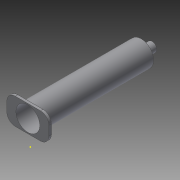
# Autodesk Inventor part: motor mount
Saved by Autodesk Inventor 2015 SP1 (Build 190203100, 203)
## iProperties
Created: 2016-07-07
Part Number: motor mount
Material: Generic
Document SubType Name: Modeling
Designer: lustinga
Density: 1 g/cm^3
Appearance: Default
Mass: 8.44804 g
Surface Area: 280.703 cm^2
Volume: 8.44804 cm^3
Author: lustinga
Autodesk Inventor part; units mm, degrees
ref_plane "YZ Plane" through (0, 0, 0) normal (1, 0, 0) x (0, 1, 0)
ref_plane "XZ Plane" through (0, 0, 0) normal (0, 1, 0) x (-1, 0, 0)
ref_plane "XY Plane" through (0, 0, 0) normal (0, 0, 1) x (1, 0, 0)
sketch "Sketch1" plane through (0, 0, 0) normal (1, 0, 0) x (0, 1, 0)
  line L0 (-81.3077, 45.4162) -> (50.6923, 45.4162)
  line L1 (56.553, 36.2588) -> (50.6923, 45.4162)
  line L2 (56.553, 36.2588) -> (63.703, 36.2588)
  line L3 (30.7678, 30.6662) -> (60.128, 30.6662)
  line L4 (63.703, 35.7588) -> (56.2794, 35.7588)
  line L5 (56.2794, 35.7588) -> (50.4187, 44.9162)
  line L6 (50.4187, 44.9162) -> (-81.3077, 44.9162)
  line L7 (63.703, 35.7588) -> (63.703, 36.2588)
  line L8 (-81.3077, 44.9162) -> (-81.3077, 45.4162)
  dimension "d26" = 132
  dimension "d29" = 7.15
  dimension "d31" = 0.5
  dimension "d38" = 29.5
  constraints: 18 end point, 3 horizontal, 2 vertical, 2 other
  measures "d26" distance of L0.start L0.end
  measures "d29" distance of L1.start L2.end
  measures "d31" distance between parallel lines of L2 L4
  measures "d38" diameter of L0 L3
revolve "Revolution1" add sketch "Sketch1" angle 360 about axis through (0, 30.7678, 30.6662) along (0, 1, 0)
sketch "Sketch2" plane through (0, -81.3077, 30.6662) normal (0, -1, 0) x (1, 0, 0)
  point P0 (0, -30.6662)
sketch "Sketch3" plane through (0, -81.3077, 30.6662) normal (0, -1, 0) x (1, 0, 0)
  line L0 (15, 15.5926) -> (-15, 15.5926)
  line L1 (-25, 5.5926) -> (-25, -5.5926)
  line L2 (-15, -15.5926) -> (15, -15.5926)
  line L3 (25, -5.5926) -> (25, 5.5926)
  arc A0 (-15, 15.5926) -> (-25, 5.5926) centre (-15, 5.5926) ccw
  arc A1 (-25, -5.5926) -> (-15, -15.5926) centre (-15, -5.5926) ccw
  arc A2 (15, -15.5926) -> (25, -5.5926) centre (15, -5.5926) ccw
  arc A3 (25, 5.5926) -> (15, 15.5926) centre (15, 5.5926) ccw
  circle A4 centre (0, 0) radius 14.25 projected
  circle A5 centre (0, 0) radius 5.0926 projected
  point P0 (0, -30.6662)
  point P1 (-25, -15.5926)
  point P2 (25, -15.5926)
  dimension "d34" = 50
  dimension "d35" = 10
  constraints: 8 end point, 8 point on circle, 8 tangent, 4 centre point, 4 point on line, 3 equal radius, 2 parallel, 1 horizontal, 1 perpendicular
  measures "d34" distance of point (25, -15.593) point (-25, -15.593)
  measures "d35" radius of A0
extrude "Extrusion2" add sketch "Sketch3" along normal blind 2.37 contours A3 L3 A2 L2 A1 L1 A0 L0
body "Solid2"
